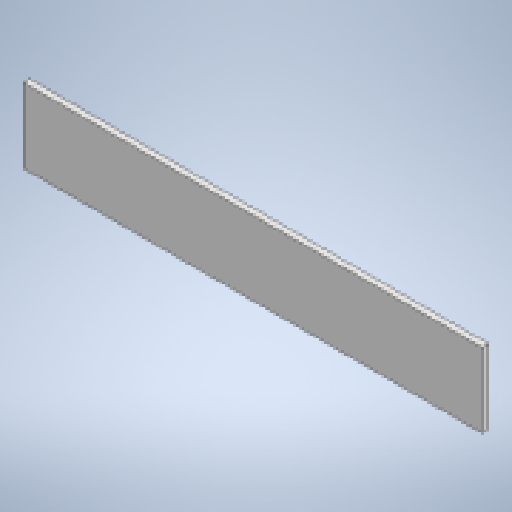
# Autodesk Inventor part: стенкаB
Saved by Autodesk Inventor 2023 (Build 270158000, 158)
## iProperties
Created: 2025-02-04
Part Number: стенкаB
Material: Типовые
Document SubType Name: Modeling
Designer: baranovaem
Density: 1 g/cm^3
Appearance: По умолчанию
Author: baranovaem
Autodesk Inventor part; units mm, degrees
ref_plane "YZ Plane" through (0, 0, 0) normal (1, 0, 0) x (0, 1, 0)
ref_plane "XZ Plane" through (0, 0, 0) normal (0, 1, 0) x (-1, 0, 0)
ref_plane "XY Plane" through (0, 0, 0) normal (0, 0, 1) x (1, 0, 0)
sketch "Эскиз1" plane through (0, 0, 0) normal (0, 0, 1) x (1, 0, 0)
  line L0 (-142.5, 23) -> (142.5, 23)
  line L1 (142.5, 23) -> (142.5, -23)
  line L2 (142.5, -23) -> (-142.5, -23)
  line L3 (-142.5, -23) -> (-142.5, 23)
  line L4 (-142.5, 23) -> (142.5, -23) construction
  line L5 (142.5, 23) -> (-142.5, -23) construction
  point P0 (0, 0)
  dimension "d0" = 285
  dimension "d1" = 46
  constraints: 12 end point, 2 midpoint, 2 parallel, 1 horizontal, 1 perpendicular
  measures "d0" distance of L1.end L2.end
  measures "d1" distance of L0.end L1.end
extrude "Выдавливание1" add sketch "Эскиз1" along normal blind 4
